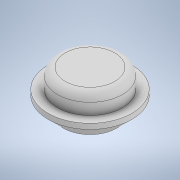
# Autodesk Inventor part: button_round
Saved by Autodesk Inventor 2022 (Build 260153000, 153)
## iProperties
Created: 2022-09-06
Part Number: button_round
Material: Generic
Document SubType Name: Modeling
Designer: simen
Density: 1 g/cm^3
Appearance: Default
Author: simen
## iProperties of the stored document button_round_3DPrint.ipt
Created: 2022-09-07
Part Number: button_round_3DPrint
Material: Generic
Document SubType Name: Modeling
Designer: simen
Density: 1 g/cm^3
Appearance: Default
Author: simen
Autodesk Inventor part; units mm, degrees
ref_plane "YZ Plane" through (0, 0, 0) normal (1, 0, 0) x (0, 1, 0)
ref_plane "XZ Plane" through (0, 0, 0) normal (0, 1, 0) x (-1, 0, 0)
ref_plane "XY Plane" through (0, 0, 0) normal (0, 0, 1) x (1, 0, 0)
sketch "Sketch1" plane through (0, 0, 0) normal (0, 1, 0) x (-1, 0, 0)
  circle A0 centre (0, 0) radius 4.25
  dimension "d0" = 8.5
  constraints: 1 centre point, 1 coincident
  measures "d0" diameter of A0
extrude "Extrusion1" add sketch "Sketch1" along normal blind 2.5
sketch "Sketch2" plane through (0, 0, 0) normal (0, -1, 0) x (1, 0, 0)
  circle A0 centre (0, 0) radius 5.5
  dimension "d3" = 11
  constraints: 1 centre point, 1 coincident
  measures "d3" diameter of A0
extrude "Extrusion2" add sketch "Sketch2" along normal blind 2.7
fillet "Fillet1" radius 1 1 edges at (4.25, 2.5, 0)
chamfer "Chamfer1" distance 2 angle 45 1 edges at (-5.5, -2.7, 0)
body "Solid1"
